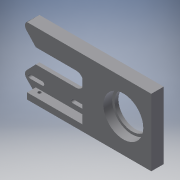
# Autodesk Inventor part: крепление подшипникового блока левая часть
Saved by Autodesk Inventor 2019.1 (Build 231200000, 200)
## iProperties
Created: 2018-08-01
Part Number: крепление подшипникового блока левая часть
Material: Типовые
Document SubType Name: Modeling
Designer: olege
Density: 1 g/cm^3
Appearance: По умолчанию
Author: olege
Autodesk Inventor part; units mm, degrees
ref_plane "YZ Plane" through (0, 0, 0) normal (1, 0, 0) x (0, 1, 0)
ref_plane "XZ Plane" through (0, 0, 0) normal (0, 1, 0) x (-1, 0, 0)
sketch "Эскиз1" plane through (0, 0, 0) normal (0, 0, 1) x (1, 0, 0)
  line L0 (50, -27) -> (-50, -27)
  line L1 (-50, -27) -> (-50, 27)
  line L2 (-50, 27) -> (50, 27)
  line L3 (50, 27) -> (50, -27)
  line L4 (50, -27) -> (-50, 27) construction
  line L5 (-50, -27) -> (50, 27) construction
  circle A0 centre (27.5, 0) radius 16.05
  point P0 (0, 0)
  point P1 (0, 0)
  dimension "d0" = 100
  dimension "d1" = 54
  dimension "d2" = 32.1
  dimension "d3" = 22.5
  constraints: 12 end point, 3 midpoint, 2 parallel, 1 centre point, 1 horizontal, 1 horizontal alignment, 1 perpendicular
  measures "d0" distance of L1.end L2.end
  measures "d1" distance of L0.end L1.end
  measures "d2" diameter of A0
  measures "d3" distance from line of L3 A0.centre
extrude "Выдавливание1" add sketch "Эскиз1" along normal blind 10
sketch "Эскиз2" plane through (0, 0, 0) normal (0, 0, -1) x (-1, 0, 0)
  circle A0 centre (-27.5, 0) radius 16.05 projected
  circle A1 centre (-27.5, 0) radius 14
  point P0 (0, 0)
  dimension "d6" = 28
  constraints: 1 centre point, 1 coincident
  measures "d6" diameter of A1
extrude "Выдавливание2" add sketch "Эскиз2" against normal blind 3
sketch "Эскиз3" plane through (0, 0, 0) normal (0, 0, -1) x (-1, 0, 0)
  circle A0 centre (-27.5, 0) radius 14 projected
  circle A1 centre (17.5, 0) radius 6
  line L0 (17.5, 6) -> (50, 6)
  line L1 (50, -27) -> (50, 27) projected
  line L2 (17.5, -6) -> (50, -6)
  line L3 (50, -6) -> (50, 6)
  point P0 (0, 0)
  dimension "d9" = 12
  dimension "d10" = 45
  constraints: 6 end point, 2 point on circle, 2 point on line, 2 tangent, 1 centre point, 1 collinear, 1 horizontal, 1 horizontal alignment, 1 parallel
  measures "d9" diameter of A1
  measures "d10" distance of A0.centre A1.centre
extrude "Выдавливание3" cut sketch "Эскиз3" against normal blind 10 contours A1 | A1 L0 L1 L2
sketch "Эскиз4" plane through (0, 0, 10) normal (0, 0, 1) x (1, 0, 0)
  line L0 (-49.5, 22) -> (-5.5, 22)
  line L1 (-5.5, 22) -> (-5.5, -22)
  line L2 (-5.5, -22) -> (-49.5, -22)
  line L3 (-49.5, -22) -> (-49.5, 22)
  line L4 (-49.5, 22) -> (-5.5, -22) construction
  line L5 (-5.5, 22) -> (-49.5, -22) construction
  arc A0 (-17.5, -6) -> (-17.5, 6) centre (-17.5, 0) ccw projected
  line L6 (-49.5, -22) -> (-62.5164, -22)
  line L7 (-62.5164, -22) -> (-62.5164, 22)
  line L8 (-62.5164, 22) -> (-49.5, 22)
  line L9 (-49.5, 22) -> (-49.5, -22)
  point P0 (0, 0)
  point P1 (-27.5, 0)
  point P2 (-27.5, 0)
  dimension "d13" = 44
  dimension "d14" = 44
  dimension "d15" = 10
  dimension "d16" = 44
  constraints: 20 end point, 4 parallel, 3 midpoint, 2 horizontal, 2 perpendicular, 1 horizontal alignment
  measures "d13" distance of L1.end L2.end
  measures "d14" distance of L0.end L1.end
  measures "d15" distance of A0.centre point (-27.5, 0)
  measures "d16" distance of L6.end L7.end
extrude "Выдавливание4" cut sketch "Эскиз4" against normal blind 7
sketch "Эскиз8" plane through (-50, -27, 10) normal (0, -1, 0) x (1, 0, 0)
  circle A0 centre (95, -5) radius 1.25
  circle A1 centre (50, -5) radius 1.25
  circle A2 centre (5, -5) radius 1.25
  line L0 (100, -10) -> (100, 0) projected
  line L1 (0, -10) -> (0, 0) projected
  line L2 (100, -10) -> (0, -10) projected
  point P0 (50, -10)
  point P1 (100, -5)
  point P2 (0, -7)
  point P3 (50, -10)
  dimension "d44" = 2.5
  dimension "d45" = 2.5
  dimension "d46" = 2.5
  dimension "d47" = 5
  dimension "d48" = 5
  constraints: 3 centre point, 3 horizontal alignment, 2 midpoint, 1 vertical alignment
  measures "d44" diameter of A0
  measures "d45" diameter of A1
  measures "d46" diameter of A2
  measures "d47" distance from line of L0 A0.centre
  measures "d48" distance from line of L1 A2.centre
extrude "Выдавливание9" cut sketch "Эскиз8" against normal up to surface (5 mm away)
sketch "Эскиз9" plane through (0, 0, 0) normal (0, 0, -1) x (-1, 0, 0)
  circle A0 centre (10.0218, 16.95) radius 1.5
  circle A1 centre (44.6782, 16.95) radius 1.5
  circle A2 centre (44.6782, -16.65) radius 1.5
  circle A3 centre (10.0218, -16.65) radius 1.5
  line L0 (-50, 27) -> (50, 27) projected
  line L1 (-50, -27) -> (-50, 27) projected
  line L2 (50, -27) -> (-50, -27) projected
  line L3 (50, -22) -> (50, -6) projected
  line L4 (50, 6) -> (50, 22) projected
  point P0 (0, 0)
  dimension "d75" = 10.05
  dimension "d76" = 60.0218
  dimension "d77" = 3
  dimension "d78" = 10.05
  dimension "d79" = 10.35
  dimension "d80" = 10.35
  dimension "d82" = 5.3218
  dimension "d83" = 3
  dimension "d84" = 3
  dimension "d85" = 3
  constraints: 4 centre point, 2 vertical alignment
  measures "d75" distance from line of L0 A0.centre
  measures "d76" distance from line of L1 A0.centre
  measures "d77" diameter of A0
  measures "d78" distance from line of L0 A1.centre
  measures "d79" distance from line of L2 A2.centre
  measures "d80" distance from line of L2 A3.centre
  measures "d82" distance from line of L4 A1.centre
  measures "d83" diameter of A3
  measures "d84" diameter of A2
  measures "d85" diameter of A1
extrude "Выдавливание10" cut sketch "Эскиз9" against normal blind 10
sketch "Эскиз10" plane through (0, 0, 0) normal (0, 0, -1) x (-1, 0, 0)
  circle A0 centre (10.0218, 16.95) radius 1.5 projected
  line L0 (10.0218, 18.45) -> (20.0218, 18.45)
  line L1 (10.0218, 15.45) -> (20.0218, 15.45)
  circle A1 centre (20.0218, 16.95) radius 1.5
  circle A2 centre (10.0218, -16.65) radius 1.5 projected
  line L2 (10.0218, -15.15) -> (20.0218, -15.15)
  line L3 (10.0218, -18.15) -> (20.0218, -18.15)
  circle A3 centre (20.0218, -16.65) radius 1.5
  line L4 (20.0218, 18.45) -> (20.0218, 15.45)
  line L5 (10.0218, 18.45) -> (10.0218, 15.45)
  line L6 (10.0218, -15.15) -> (10.0218, -18.15)
  line L7 (20.0218, -15.15) -> (20.0218, -18.15)
  point P0 (0, 0)
  dimension "d53" = 10
  dimension "d54" = 10
  dimension "d55" = 10
  dimension "d56" = 10
  constraints: 16 end point, 8 horizontal, 5 point on circle, 4 tangent, 2 vertical alignment, 1 parallel, 4 other
  measures "d53" distance of L0.start L0.end
  measures "d54" distance of L1.start L1.end
  measures "d55" distance of L2.start L2.end
  measures "d56" distance of L3.start L3.end
extrude "Выдавливание11" cut sketch "Эскиз10" against normal blind 10 contours A0 L5 | A0 L0 A1 L1 | L4 A1 | A1 L4 | A2 L2 A3 L3 | L7 A3 | A3 L7 picked at (10.3335, 17.3409)
sketch "Эскиз11" plane through (0, 0, 0) normal (0, 0, -1) x (-1, 0, 0)
  line L0 (-50, 27) -> (50, 27) projected
  line L1 (50, 6) -> (50, 27) projected
  line L2 (50, 27) -> (50, 6)
  circle A0 centre (44.6782, 16.95) radius 1.5 projected
  line L3 (44.6782, 18.45) -> (54.6782, 18.45)
  line L4 (54.6782, 18.45) -> (54.6782, 15.45)
  line L5 (54.6782, 15.45) -> (44.6782, 15.45)
  arc A1 (54.6782, 15.45) -> (54.6782, 18.45) centre (54.6782, 16.95) ccw
  arc A2 (57.6149, 14.2342) -> (57.4511, 19.8328) centre (54.6782, 16.95) ccw
  line L6 (50, 27) -> (57.4511, 19.8328)
  line L7 (50, 6) -> (57.6149, 14.2342)
  point P0 (0, 0)
  point P1 (50, 16.5)
  dimension "d60" = 10
  dimension "d61" = 3
  dimension "d62" = 8
  constraints: 12 end point, 6 point on circle, 3 tangent, 2 centre point, 2 midpoint, 2 perpendicular, 1 coincident, 1 horizontal, 1 vertical
  measures "d60" distance of L3.start L3.end
  measures "d61" distance of L3.end L4.end
  measures "d62" diameter of A2
extrude "Выдавливание12" add sketch "Эскиз11" against normal up to surface (3 mm away) contours L1 L5 A1 L3 L6 A2 L7 | L1 L3 L4 L5
extrude "Выдавливание13" cut sketch "Эскиз11" against normal blind 10 contours L5 A0 L3 L1 | L1 L3 L4 L5
ref_plane "РабПлоскость1" through (-50, 0, 0) normal (0, 1, 0) x (1, 0, 0)
sketch "Эскиз12" plane through (0, 0, 0) normal (0, 0, -1) x (-1, 0, 0)
  line L0 (50, -6) -> (17.5, -6) projected
  line L1 (50, -22) -> (50, -27) projected
  line L2 (50, -6) -> (50, -27)
  circle A0 centre (44.6782, -16.65) radius 1.5 projected
  line L3 (44.6782, -15.15) -> (54.6782, -15.15)
  line L4 (54.6782, -18.15) -> (54.6782, -15.15)
  line L5 (54.6782, -18.15) -> (44.6782, -18.15)
  circle A1 centre (54.6782, -16.65) radius 1.5
  arc A2 (57.5094, -19.4756) -> (57.5639, -13.8801) centre (54.6782, -16.65) ccw
  line L6 (50, -22) -> (50, -6) projected
  line L7 (50, -6) -> (57.5639, -13.8801)
  line L8 (50, -27) -> (57.5094, -19.4756)
  point P0 (0, 0)
  dimension "d67" = 10
  dimension "d68" = 10
  dimension "d69" = 3
  dimension "d70" = 8
  constraints: 12 end point, 4 point on circle, 4 tangent, 2 centre point, 1 coincident, 1 collinear, 1 horizontal, 1 midpoint, 1 perpendicular
  measures "d67" distance of L3.start L3.end
  measures "d68" distance of L4.start L5.end
  measures "d69" diameter of A1
  measures "d70" diameter of A2
extrude "Выдавливание14" add sketch "Эскиз12" against normal up to surface (3 mm away) contours L2 L5 A1 L3 L7 A2 L8 L1 | L2 L3 A1 L5
extrude "Выдавливание15" cut sketch "Эскиз12" against normal blind 10 contours L5 A0 L3 L2 | L2 L3 A1 L5 | A1 L4 | L4 A1
equation "\"d44\" = d45"
equation "\"d45\" = d46"
